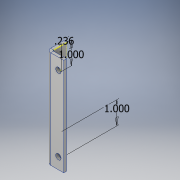
# Autodesk Inventor part: PCB_brackets
Saved by Autodesk Inventor 2017 (Build 210142000, 142)
## iProperties
Created: 2018-02-28
Part Number: PCB_brackets
Material: Aluminum 6061
Document SubType Name: Modeling
Designer: Zara
Density: 2.7 g/cm^3
Appearance: Aluminum - Flat
Sheet Metal Rule: Default
Author: Zara
Autodesk Inventor part; units mm, degrees
ref_plane "YZ Plane" through (0, 0, 0) normal (1, 0, 0) x (0, 1, 0)
ref_plane "XZ Plane" through (0, 0, 0) normal (0, 1, 0) x (-1, 0, 0)
ref_plane "XY Plane" through (0, 0, 0) normal (0, 0, 1) x (1, 0, 0)
sketch "Sketch1" plane through (0, 0, 0) normal (1, 0, 0) x (0, 1, 0)
  point P0 (0, 0)
sketch "Sketch2" plane through (0, 0, 0) normal (1, 0, 0) x (0, 1, 0)
  line L0 (-54.61, 7.9375) -> (54.61, 7.9375)
  line L1 (54.61, 7.9375) -> (54.61, -7.9375)
  line L2 (54.61, -7.9375) -> (-54.61, -7.9375)
  line L3 (-54.61, -7.9375) -> (-54.61, 7.9375)
  line L4 (-54.61, 7.9375) -> (54.61, -7.9375) construction
  line L5 (54.61, 7.9375) -> (-54.61, -7.9375) construction
  point P0 (0, 0)
  dimension "d0" = 15.875
  dimension "d1" = 109.22
  constraints: 12 end point, 2 midpoint, 2 parallel, 1 horizontal, 1 perpendicular
  measures "d0" distance of L0.end L1.end
  measures "d1" distance of L1.end L2.end
extrude "Extrusion1" add sketch "Sketch2" along normal blind 3.175
sketch "Sketch3" plane through (3.175, -54.61, 7.9375) normal (0, 0, 1) x (1, 0, 0)
  line L0 (0, 109.22) -> (0, 0)
  line L1 (0, 0) -> (15.875, 0)
  line L2 (15.875, 0) -> (15.875, 109.22)
  line L3 (15.875, 109.22) -> (0, 109.22)
  constraints: 6 end point, 1 horizontal, 1 perpendicular, 1 vertical
edge flange "Flange1" height 19.05 angle 90 thickness 3.175 bend radius 1.27 thickness toward (0, 0, 1) relief tear relief width 3.175 relief depth 1.5875 edges at (3.175, 0, 7.9375) wall of the first edge with corners at (3.175, 54.61, 7.9375) (3.175, -54.61, 7.9375) (19.05, -54.61, 7.9375) (19.05, 54.61, 7.9375)
bend "Bend1"
corner "Corner1"
sketch "Sketch4" plane through (3.175, 0, 0) normal (1, 0, 0) x (0, 0, -1)
  line L0 (1.9431, 29.21) -> (1.9431, -29.21) construction
  line L1 (7.9375, -54.61) -> (7.9375, 54.61) construction
  line L2 (7.9375, 54.61) -> (-6.6675, 54.61) projected
  line L3 (-6.6675, -54.61) -> (7.9375, -54.61) projected
  point P0 (0, 0)
  dimension "d14" = 5.9944
  dimension "d15" = 25.4
  dimension "d16" = 25.4
  constraints: 2 end point, 1 vertical
  measures "d14" distance between parallel lines of L0 L1
  measures "d15" distance from line of L0.start L2
  measures "d16" distance from line of L0.end L3
hole "Hole1" at (3.175, 29.21, -1.9431) at (3.175, -29.21, -1.9431) direction (-1, 0, 0) diameter 6 end through all
sketch "Sketch5" plane through (19.05, -54.61, 7.9375) normal (0, 0, -1) x (-1, 0, 0)
  line L0 (5.9944, 12.7) -> (5.9944, 96.52) construction
  line L1 (0, 109.22) -> (0, 0) construction
  line L2 (0, 109.22) -> (14.605, 109.22) construction
  line L3 (0, 0) -> (14.605, 0) construction
  point P0 (19.05, 54.61)
  dimension "d24" = 5.9944
  dimension "d25" = 12.7
  dimension "d26" = 12.7
  constraints: 2 end point, 1 vertical
  measures "d24" distance from line of L0.end L1
  measures "d25" distance from line of L2 L0.end
  measures "d26" distance from line of L0.start L3
hole "Hole2" at (13.0556, 41.91, 7.9375) at (13.0556, -41.91, 7.9375) direction (0, 0, 1) diameter 6 end through all
sketch "Sketch6" plane through (3.175, 0, 0) normal (1, 0, 0) x (0, 0, -1)
  circle A0 centre (1.9431, 29.21) radius 3 projected
  point P0 (0, 0)
  point P1 (4.9431, 29.21)
  constraints: 1 horizontal alignment, 1 other
equation "\"d22\" = Thickness"
equation "\"d32\" = Thickness"
equation "\"d4\" = BendReliefWidth"
equation "\"d5\" = BendReliefDepth"
equation "\"d6\" = MinimumRemnant"
equation "\"d7\" = BendRadius"
equation "\"d11\" = CornerReliefSize"
equation "\"d12\" = GapSize"
equation "\"d13\" = JacobiRadiusSize"
equation "\"BendRadius\" = Thickness"
equation "\"BendReliefWidth\" = Thickness"
equation "\"BendReliefDepth\" = 0.5 * Thickness"
equation "\"CornerReliefSize\" = 4 * Thickness"
equation "\"MinimumRemnant\" = 2 * Thickness"
equation "\"TransitionRadius\" = BendRadius"
equation "\"JacobiRadiusSize\" = BendRadius"
equation "\"GapSize\" = Thickness"
equation "\"Thickness\" = 3.175"
body "Solid1"
